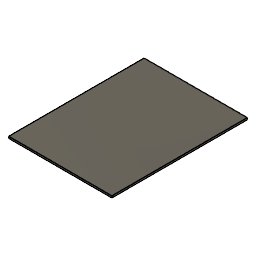
Maindarkprojectcomplete (Autodesk Fusion 360 archive; units mm, degrees)
design "pcb sketch"
part number: 2026-03-12-08-39-27-910
Autodesk Fusion 360 part; units mm, degrees
sketch "Sketch1" plane through (0, 0, 0) normal (0, 0, 1) x (1, 0, 0)
  line L0 (-24.7329, 57.4075) -> (32.4171, 57.4075)
  line L1 (32.4171, 57.4075) -> (32.4171, -17.5925)
  line L2 (32.4171, -17.5925) -> (-24.7329, -17.5925)
  line L3 (-24.7329, -17.5925) -> (-24.7329, 57.4075)
  dimension "d1" = 57.15
  dimension "d2" = 75
  constraint horizontal L0
  constraint vertical L1
  constraint horizontal L2
  constraint vertical L3
  measures "d1" distance of L0.start L0.end
  measures "d2" distance of L0 L2
extrude "Extrude1" add sketch "Sketch1" along normal blind 1

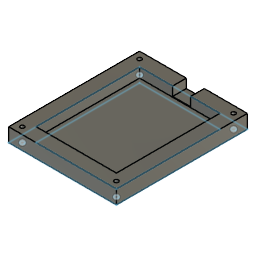
design "Darckprojectbottom"
part number: 2026-03-10-08-40-41-572
Autodesk Fusion 360 part; units mm, degrees
sketch "Sketch1" plane through (0, 0, 0) normal (0, 0, 1) x (1, 0, 0)
  line L0 (-50, 50) -> (8.2, 50)
  line L1 (8.2, 50) -> (8.2, -25)
  line L2 (8.2, -25) -> (-50, -25)
  line L3 (-50, -25) -> (-50, 50)
  line L4 (-60, 60) -> (18.2, 60)
  line L5 (18.2, 60) -> (18.2, -35)
  line L6 (18.2, -35) -> (-60, -35)
  line L7 (-60, -35) -> (-60, 60)
  circle A0 centre (-55, 55) radius 1.45
  circle A1 centre (13.2, 55) radius 1.45
  circle A2 centre (-55, -30) radius 1.45
  circle A3 centre (13.2, -30) radius 1.45
  dimension "d1" = 58.2
  dimension "d2" = 75
  dimension "d3" = 10
  dimension "d4" = 10
  dimension "d5" = 10
  dimension "d6" = 10
  dimension "d13" = 2.9
  dimension "d14" = 5
  dimension "d15" = 5
  dimension "d16" = 2.9
  dimension "d17" = 5
  dimension "d18" = 5
  dimension "d19" = 2.9
  dimension "d20" = 5
  dimension "d21" = 5
  dimension "d22" = 2.9
  dimension "d23" = 5
  dimension "d24" = 5
  constraint horizontal L0
  constraint vertical L1
  constraint horizontal L2
  constraint vertical L3
  constraint horizontal L4
  constraint vertical L5
  constraint horizontal L6
  constraint vertical L7
  measures "d1" distance of L0.start L0.end
  measures "d2" distance of L0 L2
  measures "d3" distance of L0 L4
  measures "d4" distance of L1 L5
  measures "d5" distance of L2 L6
  measures "d6" distance of L3 L7
  measures "d13" diameter of A0
  measures "d14" distance of L7 A0.centre
  measures "d15" distance of L4 A0.centre
  measures "d16" diameter of A1
  measures "d17" distance of L5 A1.centre
  measures "d18" distance of L4 A1.centre
  measures "d19" diameter of A2
  measures "d20" distance of L7 A2.centre
  measures "d21" distance of L6 A2.centre
  measures "d22" diameter of A3
  measures "d23" distance of L5 A3.centre
  measures "d24" distance of L6 A3.centre
sketch "Sketch3" plane through (0, 60, 0) normal (0, 1, 0) x (-1, 0, 0)
  line L0 (-17.15, 3) -> (60, 3)
  line L1 (60, 3) -> (60, 13)
  line L2 (60, 13) -> (-17.15, 13)
  line L3 (-17.15, 13) -> (-17.15, 3)
  line L4 (13.06, 13.5) -> (26.06, 13.5)
  line L5 (26.06, 13.5) -> (26.06, 3.5)
  line L6 (26.06, 3.5) -> (13.06, 3.5)
  line L7 (13.06, 3.5) -> (13.06, 13.5)
  dimension "d30" = 13
  dimension "d31" = 10
  dimension "d32" = 0.5
  dimension "d33" = 33.94
  constraint horizontal L4
  constraint vertical L5
  constraint horizontal L6
  constraint vertical L7
  measures "d30" distance of L4.start L4.end
  measures "d31" distance of L4 L6
  measures "d32" distance of L0 L6
  measures "d33" distance of L1 L5
extrude "Extrude7" add sketch "Sketch1" along normal blind 3 contours L0 L1 L2 L3 | L4 L5 L6 L7
extrude "Extrude8" add sketch "Sketch1" along normal blind 10
extrude "Extrude9" cut sketch "Sketch3" against normal blind 10 contours L2 L5 L6 L7

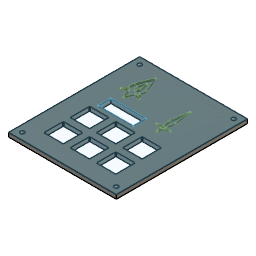
design "Darkprojectcaseupper"
part number: 2026-03-10-08-39-43-669
Autodesk Fusion 360 part; units mm, degrees
sketch "Sketch1" plane through (0, 0, 0) normal (0, 0, 1) x (1, 0, 0)
  line L0 (-36.5321, 51.7348) -> (21.6679, 51.7348)
  line L1 (21.6679, 51.7348) -> (21.6679, -23.2652)
  line L2 (21.6679, -23.2652) -> (-36.5321, -23.2652)
  line L3 (-36.5321, -23.2652) -> (-36.5321, 51.7348)
  line L4 (-46.5321, 61.894) -> (31.6679, 61.894)
  line L5 (31.6679, 61.894) -> (31.6679, -33.2652)
  line L6 (31.6679, -33.2652) -> (-46.5321, -33.2652)
  line L7 (-46.5321, -33.2652) -> (-46.5321, 61.894)
  circle A0 centre (-41.5321, -28.2652) radius 1.45
  circle A1 centre (26.6679, -28.2652) radius 1.45
  circle A2 centre (26.6679, 56.894) radius 1.45
  circle A3 centre (-41.5321, 56.894) radius 1.45
  dimension "d1" = 58.2
  dimension "d2" = 75
  dimension "d3" = 78.2
  dimension "d4" = 10
  dimension "d5" = 10
  dimension "d6" = 2.9
  dimension "d7" = 5
  dimension "d8" = 5
  dimension "d9" = 2.9
  dimension "d10" = 5
  dimension "d11" = 5
  dimension "d12" = 2.9
  dimension "d13" = 5
  dimension "d14" = 5
  dimension "d15" = 2.9
  dimension "d16" = 5
  dimension "d17" = 5
  constraint horizontal L0
  constraint vertical L1
  constraint horizontal L2
  constraint vertical L3
  constraint horizontal L4
  constraint vertical L5
  constraint horizontal L6
  constraint vertical L7
  measures "d1" distance of L0.start L0.end
  measures "d2" distance of L0 L2
  measures "d3" distance of L4.start L4.end
  measures "d4" distance of L1 L5
  measures "d5" distance of L2 L6
  measures "d6" diameter of A0
  measures "d7" distance of L6 A0.centre
  measures "d8" distance of L7 A0.centre
  measures "d9" diameter of A1
  measures "d10" distance of L5 A1.centre
  measures "d11" distance of L6 A1.centre
  measures "d12" diameter of A2
  measures "d13" distance of L5 A2.centre
  measures "d14" distance of L4 A2.centre
  measures "d15" diameter of A3
  measures "d16" distance of L4 A3.centre
  measures "d17" distance of L7 A3.centre
extrude "Extrude1" add sketch "Sketch1" along normal blind 3 contours L0 L1 L2 L3 | L4 L5 L6 L7
sketch "plate-2026-03-10T08_09_48.160Z" plane through (0, 0, 3) normal (0, 0, 1) x (1, 0, 0)
  line L0 (-13.925, 12.475) -> (-0.925, 12.475)
  line L1 (-13.925, -1.525) -> (-0.925, -1.525)
  line L2 (-14.425, 11.975) -> (-14.425, -1.025)
  line L3 (-0.425, 11.975) -> (-0.425, -1.025)
  arc A0 (-13.925, 12.475) -> (-14.425, 11.975) centre (-13.925, 11.975) ccw
  arc A1 (-0.425, 11.975) -> (-0.925, 12.475) centre (-0.925, 11.975) ccw
  arc A2 (-14.425, -1.025) -> (-13.925, -1.525) centre (-13.925, -1.025) ccw
  arc A3 (-0.925, -1.525) -> (-0.425, -1.025) centre (-0.925, -1.025) ccw
  line L4 (5.125, 12.475) -> (18.125, 12.475)
  line L5 (5.125, -1.525) -> (18.125, -1.525)
  line L6 (4.625, 11.975) -> (4.625, -1.025)
  line L7 (18.625, 11.975) -> (18.625, -1.025)
  arc A4 (5.125, 12.475) -> (4.625, 11.975) centre (5.125, 11.975) ccw
  arc A5 (18.625, 11.975) -> (18.125, 12.475) centre (18.125, 11.975) ccw
  arc A6 (4.625, -1.025) -> (5.125, -1.525) centre (5.125, -1.025) ccw
  arc A7 (18.125, -1.525) -> (18.625, -1.025) centre (18.125, -1.025) ccw
  line L8 (-32.975, -6.575) -> (-19.975, -6.575)
  line L9 (-32.975, -20.575) -> (-19.975, -20.575)
  line L10 (-33.475, -7.075) -> (-33.475, -20.075)
  line L11 (-19.475, -7.075) -> (-19.475, -20.075)
  arc A8 (-32.975, -6.575) -> (-33.475, -7.075) centre (-32.975, -7.075) ccw
  arc A9 (-19.475, -7.075) -> (-19.975, -6.575) centre (-19.975, -7.075) ccw
  arc A10 (-33.475, -20.075) -> (-32.975, -20.575) centre (-32.975, -20.075) ccw
  arc A11 (-19.975, -20.575) -> (-19.475, -20.075) centre (-19.975, -20.075) ccw
  line L12 (-13.925, -6.575) -> (-0.925, -6.575)
  line L13 (-13.925, -20.575) -> (-0.925, -20.575)
  line L14 (-14.425, -7.075) -> (-14.425, -20.075)
  line L15 (-0.425, -7.075) -> (-0.425, -20.075)
  arc A12 (-13.925, -6.575) -> (-14.425, -7.075) centre (-13.925, -7.075) ccw
  arc A13 (-0.425, -7.075) -> (-0.925, -6.575) centre (-0.925, -7.075) ccw
  arc A14 (-14.425, -20.075) -> (-13.925, -20.575) centre (-13.925, -20.075) ccw
  arc A15 (-0.925, -20.575) -> (-0.425, -20.075) centre (-0.925, -20.075) ccw
  line L16 (5.125, -6.575) -> (18.125, -6.575)
  line L17 (5.125, -20.575) -> (18.125, -20.575)
  line L18 (4.625, -7.075) -> (4.625, -20.075)
  line L19 (18.625, -7.075) -> (18.625, -20.075)
  arc A16 (5.125, -6.575) -> (4.625, -7.075) centre (5.125, -7.075) ccw
  arc A17 (18.625, -7.075) -> (18.125, -6.575) centre (18.125, -7.075) ccw
  arc A18 (4.625, -20.075) -> (5.125, -20.575) centre (5.125, -20.075) ccw
  arc A19 (18.125, -20.575) -> (18.625, -20.075) centre (18.125, -20.075) ccw
  line L20 (-36, -23.1) -> (21.15, -23.1)
  line L21 (-36, 15) -> (21.15, 15)
  line L22 (-36, -23.1) -> (-36, 15)
  line L23 (21.15, -23.1) -> (21.15, 15)
extrude "Extrude2" cut sketch "plate-2026-03-10T08_09_48.160Z" against normal blind 3 contours L0 L1 L2 L3 A0 A1 A2 A3 | L4 L5 L6 L7 A4 A5 A6 A7 | L8 L9 L10 L11 A8 A9 A10 A11 | L12 L13 L14 L15 A12 A13 A14 A15 | L16 L17 L18 L19 A16 A17 A18 A19
sketch "plate-2026-03-10T20_02_18.026Z" plane through (0, 0, 3) normal (0, 0, 1) x (1, 0, 0)
  line L0 (-32.975, 12.475) -> (-19.975, 12.475)
  line L1 (-32.975, -1.525) -> (-19.975, -1.525)
  line L2 (-33.475, 11.975) -> (-33.475, -1.025)
  line L3 (-19.475, 11.975) -> (-19.475, -1.025)
  arc A0 (-32.975, 12.475) -> (-33.475, 11.975) centre (-32.975, 11.975) ccw
  arc A1 (-19.475, 11.975) -> (-19.975, 12.475) centre (-19.975, 11.975) ccw
  arc A2 (-33.475, -1.025) -> (-32.975, -1.525) centre (-32.975, -1.025) ccw
  arc A3 (-19.975, -1.525) -> (-19.475, -1.025) centre (-19.975, -1.025) ccw
  line L4 (-13.925, 12.475) -> (-0.925, 12.475)
  line L5 (-13.925, -1.525) -> (-0.925, -1.525)
  line L6 (-14.425, 11.975) -> (-14.425, -1.025)
  line L7 (-0.425, 11.975) -> (-0.425, -1.025)
  arc A4 (-13.925, 12.475) -> (-14.425, 11.975) centre (-13.925, 11.975) ccw
  arc A5 (-0.425, 11.975) -> (-0.925, 12.475) centre (-0.925, 11.975) ccw
  arc A6 (-14.425, -1.025) -> (-13.925, -1.525) centre (-13.925, -1.025) ccw
  arc A7 (-0.925, -1.525) -> (-0.425, -1.025) centre (-0.925, -1.025) ccw
  line L8 (5.125, 12.475) -> (18.125, 12.475)
  line L9 (5.125, -1.525) -> (18.125, -1.525)
  line L10 (4.625, 11.975) -> (4.625, -1.025)
  line L11 (18.625, 11.975) -> (18.625, -1.025)
  arc A8 (5.125, 12.475) -> (4.625, 11.975) centre (5.125, 11.975) ccw
  arc A9 (18.625, 11.975) -> (18.125, 12.475) centre (18.125, 11.975) ccw
  arc A10 (4.625, -1.025) -> (5.125, -1.525) centre (5.125, -1.025) ccw
  arc A11 (18.125, -1.525) -> (18.625, -1.025) centre (18.125, -1.025) ccw
  line L12 (-32.975, -6.575) -> (-19.975, -6.575)
  line L13 (-32.975, -20.575) -> (-19.975, -20.575)
  line L14 (-33.475, -7.075) -> (-33.475, -20.075)
  line L15 (-19.475, -7.075) -> (-19.475, -20.075)
  arc A12 (-32.975, -6.575) -> (-33.475, -7.075) centre (-32.975, -7.075) ccw
  arc A13 (-19.475, -7.075) -> (-19.975, -6.575) centre (-19.975, -7.075) ccw
  arc A14 (-33.475, -20.075) -> (-32.975, -20.575) centre (-32.975, -20.075) ccw
  arc A15 (-19.975, -20.575) -> (-19.475, -20.075) centre (-19.975, -20.075) ccw
  line L16 (-13.925, -6.575) -> (-0.925, -6.575)
  line L17 (-13.925, -20.575) -> (-0.925, -20.575)
  line L18 (-14.425, -7.075) -> (-14.425, -20.075)
  line L19 (-0.425, -7.075) -> (-0.425, -20.075)
  arc A16 (-13.925, -6.575) -> (-14.425, -7.075) centre (-13.925, -7.075) ccw
  arc A17 (-0.425, -7.075) -> (-0.925, -6.575) centre (-0.925, -7.075) ccw
  arc A18 (-14.425, -20.075) -> (-13.925, -20.575) centre (-13.925, -20.075) ccw
  arc A19 (-0.925, -20.575) -> (-0.425, -20.075) centre (-0.925, -20.075) ccw
  line L20 (5.125, -6.575) -> (18.125, -6.575)
  line L21 (5.125, -20.575) -> (18.125, -20.575)
  line L22 (4.625, -7.075) -> (4.625, -20.075)
  line L23 (18.625, -7.075) -> (18.625, -20.075)
  arc A20 (5.125, -6.575) -> (4.625, -7.075) centre (5.125, -7.075) ccw
  arc A21 (18.625, -7.075) -> (18.125, -6.575) centre (18.125, -7.075) ccw
  arc A22 (4.625, -20.075) -> (5.125, -20.575) centre (5.125, -20.075) ccw
  arc A23 (18.125, -20.575) -> (18.625, -20.075) centre (18.125, -20.075) ccw
  line L24 (-36, -23.1) -> (21.15, -23.1)
  line L25 (-36, 15) -> (21.15, 15)
  line L26 (-36, -23.1) -> (-36, 15)
  line L27 (21.15, -23.1) -> (21.15, 15)
extrude "Extrude3" cut sketch "plate-2026-03-10T20_02_18.026Z" against normal blind 3 contours L0 L1 L2 L3 A0 A1 A2 A3
sketch "Sketch6" plane through (0, 0, 3) normal (0, 0, 1) x (-1, 0, 0)
  line L0 (33.475, 1.025) -> (33.475, -11.975)
  arc A0 (32.975, -12.475) -> (33.475, -11.975) centre (32.975, -11.975) ccw
  line L1 (32.975, -12.475) -> (19.975, -12.475)
  arc A1 (19.475, -11.975) -> (19.975, -12.475) centre (19.975, -11.975) ccw
  line L2 (19.475, -11.975) -> (19.475, 1.025)
  arc A2 (19.975, 1.525) -> (19.475, 1.025) centre (19.975, 1.025) ccw
  line L3 (19.975, 1.525) -> (32.975, 1.525)
  arc A3 (33.475, 1.025) -> (32.975, 1.525) centre (32.975, 1.025) ccw
  line L4 (-4.625, 20.075) -> (-4.625, 7.075)
  arc A4 (-5.125, 6.575) -> (-4.625, 7.075) centre (-5.125, 7.075) ccw
  line L5 (-5.125, 6.575) -> (-18.125, 6.575)
  arc A5 (-18.625, 7.075) -> (-18.125, 6.575) centre (-18.125, 7.075) ccw
  line L6 (-18.625, 7.075) -> (-18.625, 20.075)
  arc A6 (-18.125, 20.575) -> (-18.625, 20.075) centre (-18.125, 20.075) ccw
  line L7 (-18.125, 20.575) -> (-5.125, 20.575)
  arc A7 (-4.625, 20.075) -> (-5.125, 20.575) centre (-5.125, 20.075) ccw
  line L8 (-4.625, 1.025) -> (-4.625, -11.975)
  arc A8 (-5.125, -12.475) -> (-4.625, -11.975) centre (-5.125, -11.975) ccw
  line L9 (-5.125, -12.475) -> (-18.125, -12.475)
  arc A9 (-18.625, -11.975) -> (-18.125, -12.475) centre (-18.125, -11.975) ccw
  line L10 (-18.625, -11.975) -> (-18.625, 1.025)
  arc A10 (-18.125, 1.525) -> (-18.625, 1.025) centre (-18.125, 1.025) ccw
  line L11 (-18.125, 1.525) -> (-5.125, 1.525)
  arc A11 (-4.625, 1.025) -> (-5.125, 1.525) centre (-5.125, 1.025) ccw
  line L12 (14.425, 20.075) -> (14.425, 7.075)
  arc A12 (13.925, 6.575) -> (14.425, 7.075) centre (13.925, 7.075) ccw
  line L13 (13.925, 6.575) -> (0.925, 6.575)
  arc A13 (0.425, 7.075) -> (0.925, 6.575) centre (0.925, 7.075) ccw
  line L14 (0.425, 7.075) -> (0.425, 20.075)
  arc A14 (0.925, 20.575) -> (0.425, 20.075) centre (0.925, 20.075) ccw
  line L15 (0.925, 20.575) -> (13.925, 20.575)
  arc A15 (14.425, 20.075) -> (13.925, 20.575) centre (13.925, 20.075) ccw
  line L16 (14.425, 1.025) -> (14.425, -11.975)
  arc A16 (13.925, -12.475) -> (14.425, -11.975) centre (13.925, -11.975) ccw
  line L17 (13.925, -12.475) -> (0.925, -12.475)
  arc A17 (0.425, -11.975) -> (0.925, -12.475) centre (0.925, -11.975) ccw
  line L18 (0.425, -11.975) -> (0.425, 1.025)
  arc A18 (0.925, 1.525) -> (0.425, 1.025) centre (0.925, 1.025) ccw
  line L19 (0.925, 1.525) -> (13.925, 1.525)
  arc A19 (14.425, 1.025) -> (13.925, 1.525) centre (13.925, 1.025) ccw
  line L20 (33.475, 20.075) -> (33.475, 7.075)
  arc A20 (32.975, 6.575) -> (33.475, 7.075) centre (32.975, 7.075) ccw
  line L21 (32.975, 6.575) -> (19.975, 6.575)
  arc A21 (19.475, 7.075) -> (19.975, 6.575) centre (19.975, 7.075) ccw
  line L22 (19.475, 7.075) -> (19.475, 20.075)
  arc A22 (19.975, 20.575) -> (19.475, 20.075) centre (19.975, 20.075) ccw
  line L23 (19.975, 20.575) -> (32.975, 20.575)
  arc A23 (33.475, 20.075) -> (32.975, 20.575) centre (32.975, 20.075) ccw
  circle A24 centre (-26.6679, 28.2652) radius 1.45
  circle A25 centre (41.5321, -56.894) radius 1.45
  circle A26 centre (41.5321, 28.2652) radius 1.45
  circle A27 centre (-26.6679, -56.894) radius 1.45
  line L24 (46.5321, 33.2652) -> (-31.6679, 33.2652)
  line L25 (-31.6679, 33.2652) -> (-31.6679, -61.894)
  line L26 (-31.6679, -61.894) -> (46.5321, -61.894)
  line L27 (46.5321, -61.894) -> (46.5321, 33.2652)
  line L28 (30.5252, -25) -> (5.2252, -25)
  line L29 (5.2252, -25) -> (5.2252, -15.9341)
  line L30 (5.2252, -15.9341) -> (30.5252, -15.9341)
  line L31 (30.5252, -15.9341) -> (30.5252, -25)
  dimension "d28" = 25.3
  constraint horizontal L28
  constraint vertical L29
  constraint horizontal L30
  constraint vertical L31
  measures "d28" distance of L28.start L28.end
extrude "Extrude5" cut sketch "Sketch6" against normal blind 3 contours L28 L29 L30 L31
sketch "Sketch7" plane through (0, 0, 3) normal (0, 0, 1) x (-1, 0, 0)
  line L0 (5.2252, -25) -> (5.2252, -15.9341)
  line L1 (5.2252, -15.9341) -> (30.5252, -15.9341)
  line L2 (30.5252, -15.9341) -> (30.5252, -25)
  line L3 (30.5252, -25) -> (5.2252, -25)
  line L4 (33.475, 1.025) -> (33.475, -11.975)
  arc A0 (32.975, -12.475) -> (33.475, -11.975) centre (32.975, -11.975) ccw
  line L5 (32.975, -12.475) -> (19.975, -12.475)
  arc A1 (19.475, -11.975) -> (19.975, -12.475) centre (19.975, -11.975) ccw
  line L6 (19.475, -11.975) -> (19.475, 1.025)
  arc A2 (19.975, 1.525) -> (19.475, 1.025) centre (19.975, 1.025) ccw
  line L7 (19.975, 1.525) -> (32.975, 1.525)
  arc A3 (33.475, 1.025) -> (32.975, 1.525) centre (32.975, 1.025) ccw
  line L8 (-4.625, 20.075) -> (-4.625, 7.075)
  arc A4 (-5.125, 6.575) -> (-4.625, 7.075) centre (-5.125, 7.075) ccw
  line L9 (-5.125, 6.575) -> (-18.125, 6.575)
  arc A5 (-18.625, 7.075) -> (-18.125, 6.575) centre (-18.125, 7.075) ccw
  line L10 (-18.625, 7.075) -> (-18.625, 20.075)
  arc A6 (-18.125, 20.575) -> (-18.625, 20.075) centre (-18.125, 20.075) ccw
  line L11 (-18.125, 20.575) -> (-5.125, 20.575)
  arc A7 (-4.625, 20.075) -> (-5.125, 20.575) centre (-5.125, 20.075) ccw
  line L12 (-4.625, 1.025) -> (-4.625, -11.975)
  arc A8 (-5.125, -12.475) -> (-4.625, -11.975) centre (-5.125, -11.975) ccw
  line L13 (-5.125, -12.475) -> (-18.125, -12.475)
  arc A9 (-18.625, -11.975) -> (-18.125, -12.475) centre (-18.125, -11.975) ccw
  line L14 (-18.625, -11.975) -> (-18.625, 1.025)
  arc A10 (-18.125, 1.525) -> (-18.625, 1.025) centre (-18.125, 1.025) ccw
  line L15 (-18.125, 1.525) -> (-5.125, 1.525)
  arc A11 (-4.625, 1.025) -> (-5.125, 1.525) centre (-5.125, 1.025) ccw
  line L16 (14.425, 20.075) -> (14.425, 7.075)
  arc A12 (13.925, 6.575) -> (14.425, 7.075) centre (13.925, 7.075) ccw
  line L17 (13.925, 6.575) -> (0.925, 6.575)
  arc A13 (0.425, 7.075) -> (0.925, 6.575) centre (0.925, 7.075) ccw
  line L18 (0.425, 7.075) -> (0.425, 20.075)
  arc A14 (0.925, 20.575) -> (0.425, 20.075) centre (0.925, 20.075) ccw
  line L19 (0.925, 20.575) -> (13.925, 20.575)
  arc A15 (14.425, 20.075) -> (13.925, 20.575) centre (13.925, 20.075) ccw
  line L20 (14.425, 1.025) -> (14.425, -11.975)
  arc A16 (13.925, -12.475) -> (14.425, -11.975) centre (13.925, -11.975) ccw
  line L21 (13.925, -12.475) -> (0.925, -12.475)
  arc A17 (0.425, -11.975) -> (0.925, -12.475) centre (0.925, -11.975) ccw
  line L22 (0.425, -11.975) -> (0.425, 1.025)
  arc A18 (0.925, 1.525) -> (0.425, 1.025) centre (0.925, 1.025) ccw
  line L23 (0.925, 1.525) -> (13.925, 1.525)
  arc A19 (14.425, 1.025) -> (13.925, 1.525) centre (13.925, 1.025) ccw
  line L24 (33.475, 20.075) -> (33.475, 7.075)
  arc A20 (32.975, 6.575) -> (33.475, 7.075) centre (32.975, 7.075) ccw
  line L25 (32.975, 6.575) -> (19.975, 6.575)
  arc A21 (19.475, 7.075) -> (19.975, 6.575) centre (19.975, 7.075) ccw
  line L26 (19.475, 7.075) -> (19.475, 20.075)
  arc A22 (19.975, 20.575) -> (19.475, 20.075) centre (19.975, 20.075) ccw
  line L27 (19.975, 20.575) -> (32.975, 20.575)
  arc A23 (33.475, 20.075) -> (32.975, 20.575) centre (32.975, 20.075) ccw
  circle A24 centre (-26.6679, 28.2652) radius 1.45
  circle A25 centre (41.5321, -56.894) radius 1.45
  circle A26 centre (41.5321, 28.2652) radius 1.45
  circle A27 centre (-26.6679, -56.894) radius 1.45
  line L28 (46.5321, 33.2652) -> (-31.6679, 33.2652)
  line L29 (-31.6679, 33.2652) -> (-31.6679, -61.894)
  line L30 (-31.6679, -61.894) -> (46.5321, -61.894)
  line L31 (46.5321, -61.894) -> (46.5321, 33.2652)
  line L32 (-6.7708, -21.3229) -> (-5.7125, -24.7625)
  line L33 (-5.7125, -24.7625) -> (-2.0083, -25.8208)
  line L34 (-2.0083, -25.8208) -> (-5.7125, -26.8792)
  line L35 (-5.7125, -26.8792) -> (-4.9187, -32.7)
  line L36 (-4.9187, -32.7) -> (-6.7708, -45.1354)
  line L37 (-6.7708, -45.1354) -> (-8.6229, -32.7)
  line L38 (-8.6229, -32.7) -> (-7.8292, -26.8792)
  line L39 (-7.8292, -26.8792) -> (-11.5333, -25.8208)
  line L40 (-11.5333, -25.8208) -> (-7.8292, -24.7625)
  line L41 (-7.8292, -24.7625) -> (-6.7708, -21.3229)
extrude "Extrude6" cut sketch "Sketch7" against normal blind 0.5 contours L32 L33 L34 L35 L36 L37 L38 L39 L40 L41
sketch "Sketch8" plane through (0, 0, 3) normal (0, 0, 1) x (-1, 0, 0)
  line L0 (-7.8292, -26.8792) -> (-11.5333, -25.8208)
  line L1 (-11.5333, -25.8208) -> (-7.8292, -24.7625)
  line L2 (-7.8292, -24.7625) -> (-6.7708, -21.3229)
  line L3 (-6.7708, -21.3229) -> (-5.7125, -24.7625)
  line L4 (-5.7125, -24.7625) -> (-2.0083, -25.8208)
  line L5 (-2.0083, -25.8208) -> (-5.7125, -26.8792)
  line L6 (-5.7125, -26.8792) -> (-4.9187, -32.7)
  line L7 (-4.9187, -32.7) -> (-6.7708, -45.1354)
  line L8 (-6.7708, -45.1354) -> (-8.6229, -32.7)
  line L9 (-8.6229, -32.7) -> (-7.8292, -26.8792)
  line L10 (5.2252, -25) -> (5.2252, -15.9341)
  line L11 (5.2252, -15.9341) -> (30.5252, -15.9341)
  line L12 (30.5252, -15.9341) -> (30.5252, -25)
  line L13 (30.5252, -25) -> (5.2252, -25)
  line L14 (33.475, 1.025) -> (33.475, -11.975)
  arc A0 (32.975, -12.475) -> (33.475, -11.975) centre (32.975, -11.975) ccw
  line L15 (32.975, -12.475) -> (19.975, -12.475)
  arc A1 (19.475, -11.975) -> (19.975, -12.475) centre (19.975, -11.975) ccw
  line L16 (19.475, -11.975) -> (19.475, 1.025)
  arc A2 (19.975, 1.525) -> (19.475, 1.025) centre (19.975, 1.025) ccw
  line L17 (19.975, 1.525) -> (32.975, 1.525)
  arc A3 (33.475, 1.025) -> (32.975, 1.525) centre (32.975, 1.025) ccw
  line L18 (-4.625, 20.075) -> (-4.625, 7.075)
  arc A4 (-5.125, 6.575) -> (-4.625, 7.075) centre (-5.125, 7.075) ccw
  line L19 (-5.125, 6.575) -> (-18.125, 6.575)
  arc A5 (-18.625, 7.075) -> (-18.125, 6.575) centre (-18.125, 7.075) ccw
  line L20 (-18.625, 7.075) -> (-18.625, 20.075)
  arc A6 (-18.125, 20.575) -> (-18.625, 20.075) centre (-18.125, 20.075) ccw
  line L21 (-18.125, 20.575) -> (-5.125, 20.575)
  arc A7 (-4.625, 20.075) -> (-5.125, 20.575) centre (-5.125, 20.075) ccw
  line L22 (-4.625, 1.025) -> (-4.625, -11.975)
  arc A8 (-5.125, -12.475) -> (-4.625, -11.975) centre (-5.125, -11.975) ccw
  line L23 (-5.125, -12.475) -> (-18.125, -12.475)
  arc A9 (-18.625, -11.975) -> (-18.125, -12.475) centre (-18.125, -11.975) ccw
  line L24 (-18.625, -11.975) -> (-18.625, 1.025)
  arc A10 (-18.125, 1.525) -> (-18.625, 1.025) centre (-18.125, 1.025) ccw
  line L25 (-18.125, 1.525) -> (-5.125, 1.525)
  arc A11 (-4.625, 1.025) -> (-5.125, 1.525) centre (-5.125, 1.025) ccw
  line L26 (14.425, 20.075) -> (14.425, 7.075)
  arc A12 (13.925, 6.575) -> (14.425, 7.075) centre (13.925, 7.075) ccw
  line L27 (13.925, 6.575) -> (0.925, 6.575)
  arc A13 (0.425, 7.075) -> (0.925, 6.575) centre (0.925, 7.075) ccw
  line L28 (0.425, 7.075) -> (0.425, 20.075)
  arc A14 (0.925, 20.575) -> (0.425, 20.075) centre (0.925, 20.075) ccw
  line L29 (0.925, 20.575) -> (13.925, 20.575)
  arc A15 (14.425, 20.075) -> (13.925, 20.575) centre (13.925, 20.075) ccw
  line L30 (14.425, 1.025) -> (14.425, -11.975)
  arc A16 (13.925, -12.475) -> (14.425, -11.975) centre (13.925, -11.975) ccw
  line L31 (13.925, -12.475) -> (0.925, -12.475)
  arc A17 (0.425, -11.975) -> (0.925, -12.475) centre (0.925, -11.975) ccw
  line L32 (0.425, -11.975) -> (0.425, 1.025)
  arc A18 (0.925, 1.525) -> (0.425, 1.025) centre (0.925, 1.025) ccw
  line L33 (0.925, 1.525) -> (13.925, 1.525)
  arc A19 (14.425, 1.025) -> (13.925, 1.525) centre (13.925, 1.025) ccw
  line L34 (33.475, 20.075) -> (33.475, 7.075)
  arc A20 (32.975, 6.575) -> (33.475, 7.075) centre (32.975, 7.075) ccw
  line L35 (32.975, 6.575) -> (19.975, 6.575)
  arc A21 (19.475, 7.075) -> (19.975, 6.575) centre (19.975, 7.075) ccw
  line L36 (19.475, 7.075) -> (19.475, 20.075)
  arc A22 (19.975, 20.575) -> (19.475, 20.075) centre (19.975, 20.075) ccw
  line L37 (19.975, 20.575) -> (32.975, 20.575)
  arc A23 (33.475, 20.075) -> (32.975, 20.575) centre (32.975, 20.075) ccw
  circle A24 centre (-26.6679, 28.2652) radius 1.45
  circle A25 centre (41.5321, -56.894) radius 1.45
  circle A26 centre (41.5321, 28.2652) radius 1.45
  circle A27 centre (-26.6679, -56.894) radius 1.45
  line L38 (46.5321, 33.2652) -> (-31.6679, 33.2652)
  line L39 (-31.6679, 33.2652) -> (-31.6679, -61.894)
  line L40 (-31.6679, -61.894) -> (46.5321, -61.894)
  line L41 (46.5321, -61.894) -> (46.5321, 33.2652)
  spline S0 degree 3 poles (26.7708, -53.6771) (28.3583, -50.2375) (29.9458, -46.5333) (31.0042, -43.0937) knots 0 0 0 0 1 1 1 1
  spline S1 degree 3 poles (31.0042, -43.0937) (31.5333, -41.2417) (31.5333, -39.6542) (30.7396, -38.3312) knots 0 0 0 0 1 1 1 1
  line L42 (30.7396, -38.3312) -> (33.3854, -35.1562)
  line L43 (33.3854, -35.1562) -> (29.4167, -36.4792)
  spline S2 degree 3 poles (29.4167, -36.4792) (28.3583, -34.3625) (27.5646, -32.5104) (26.7708, -30.6583) knots 0 0 0 0 1 1 1 1
  spline S3 degree 3 poles (26.7708, -30.6583) (25.9771, -32.5104) (25.1833, -34.3625) (24.125, -36.4792) knots 0 0 0 0 1 1 1 1
  line L44 (24.125, -36.4792) -> (20.1563, -35.1562)
  line L45 (20.1563, -35.1562) -> (22.8021, -38.3312)
  spline S4 degree 3 poles (22.8021, -38.3312) (22.0083, -39.6542) (22.0083, -41.2417) (22.5375, -43.0937) knots 0 0 0 0 1 1 1 1
  spline S5 degree 3 poles (22.5375, -43.0937) (23.5958, -46.5333) (25.1833, -50.2375) (26.7708, -53.6771) knots 0 0 0 0 1 1 1 1
  spline S6 degree 3 poles (26.7708, -47.0625) (25.9771, -44.9458) (25.4479, -43.0937) (25.4479, -41.7708) knots 0 0 0 0 1 1 1 1
  spline S7 degree 3 poles (25.4479, -41.7708) (25.4479, -40.4479) (25.9771, -39.6542) (26.7708, -39.125) knots 0 0 0 0 1 1 1 1
  spline S8 degree 3 poles (26.7708, -39.125) (27.5646, -39.6542) (28.0938, -40.4479) (28.0938, -41.7708) knots 0 0 0 0 1 1 1 1
  spline S9 degree 3 poles (28.0938, -41.7708) (28.0938, -43.0937) (27.5646, -44.9458) (26.7708, -47.0625) knots 0 0 0 0 1 1 1 1
extrude "Extrude7" cut sketch "Sketch8" against normal blind 0.5 contours S0 S1 L42 L43 S2 S3 L44 L45 S4 S5

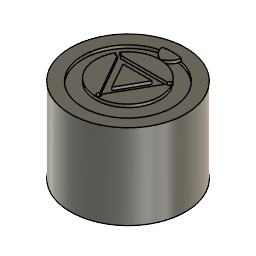
design "Untitled"
part number: 2026-03-13-09-33-52-471
Autodesk Fusion 360 part; units mm, degrees
sketch "Sketch1" plane through (0, 0, 0) normal (0, 0, 1) x (1, 0, 0)
  circle A0 centre (38.1204, 22.2369) radius 9.5
  dimension "d1" = 19
  measures "d1" diameter of A0
extrude "Extrude1" add sketch "Sketch1" along normal blind 14 makes body 1
sketch "Sketch3" plane through (0, 0, 0) normal (0, 0, 1) x (1, 0, 0)
  arc A0 (38.353, 24.7546) -> (40.7938, 22.3138) centre (38.353, 22.3138) cw
  arc A1 (40.7938, 22.3138) -> (38.353, 19.873) centre (38.353, 22.3138) cw
  line L0 (38.353, 19.873) -> (35.9122, 19.873)
  line L1 (35.9122, 19.873) -> (35.9122, 24.7546)
  line L2 (35.9122, 24.7546) -> (38.353, 24.7546)
extrude "Extrude2" cut sketch "Sketch3" along normal blind 10 bodies 1
sketch "Sketch4" plane through (0, 0, 14) normal (0, 0, 1) x (-1, 0, 0)
  circle A0 centre (-38.1204, -22.2369) radius 9.5
  circle A1 centre (-38.201, -22.1343) radius 7.4083
  circle A2 centre (-38.201, -22.1343) radius 5.2917
  line L0 (-38.201, -17.3718) -> (-33.9677, -24.7801)
  line L1 (-33.9677, -24.7801) -> (-42.4344, -24.7801)
  line L2 (-42.4344, -24.7801) -> (-38.201, -17.3718)
  line L3 (-38.201, -19.4884) -> (-35.8198, -23.7218)
  line L4 (-35.8198, -23.7218) -> (-40.5823, -23.7218)
  line L5 (-40.5823, -23.7218) -> (-38.201, -19.4884)
  line L6 (-38.201, -14.7259) -> (-38.201, -29.5426)
  line L7 (-45.6094, -22.1343) -> (-30.7927, -22.1343)
  line L8 (-40.8469, -16.3134) -> (-42.4344, -15.2551)
  line L9 (-35.5552, -16.3134) -> (-33.9677, -15.2551)
  spline S0 degree 3 poles (-38.201, -27.4259) (-37.1427, -27.9551) (-36.6135, -28.7488) (-36.6135, -29.5426) knots 0 0 0 0 1 1 1 1
  spline S1 degree 3 poles (-38.201, -27.4259) (-39.2594, -27.9551) (-39.7885, -28.7488) (-39.7885, -29.5426) knots 0 0 0 0 1 1 1 1
  circle A3 centre (-42.4344, -24.7801) radius 0.3704
  circle A4 centre (-33.9677, -24.7801) radius 0.3704
  circle A5 centre (-38.201, -17.3718) radius 0.3704
  point P0 (-32.9094, -22.1343)
  point P1 (-42.064, -24.7801)
  point P2 (-33.5973, -24.7801)
  point P3 (-37.8306, -17.3718)
extrude "Extrude3" cut sketch "Sketch4" against normal blind 0.5 contours A1 A2 L6 L7 | A1 A2 L7 S0 A4 | A1 L6 S0 | A2 L0 L6 L7 A5 | A2 L0 L7 A4 | A1 A2 L6 L7 | A1 L6 S1 | A1 A2 L7 S1 A3 | A2 L1 L6 A4 | A2 L1 L6 A3 | A2 L2 L6 L7 A5 | A2 A4 | A2 L0 L1 A4 | L0 L3 L6 L7 A5 | L0 L1 L3 L4 L6 L7 A4 | A2 A3 | A2 L1 L2 A3 | L1 L2 L4 L5 L6 L7 A3 | A2 L2 L7 A3 | L0 L6 A5 | L2 L6 A5 | L0 L1 A4 | L0 L6 A5 | L3 L6 L7 | L3 L4 L6 L7 | L1 L2 A3 | L4 L5 L6 L7 | L2 L5 L6 L7 A5 | L2 L6 A5 | L5 L6 L7 bodies 1
extrude "Extrude4" add sketch "Sketch4" along normal blind 0.5 separate body contours L3 L6 L7 | L3 L4 L6 L7 | L4 L5 L6 L7 | L5 L6 L7 makes body 2
extrude "Extrude5" add sketch "Sketch4" along normal blind 0.5 separate body contours A2 L0 L6 L7 A5 | A2 L0 L7 A4 | A2 L1 L6 A4 | A2 L1 L6 A3 | A2 L2 L6 L7 A5 | A2 L2 L7 A3 makes body 3 at (38.3325, 25.6571, 14) makes body 4 at (41.2514, 20.7773, 14.5)
extrude "Extrude6" add sketch "Sketch4" along normal blind 0.5 contours A1 L6 S0 | A1 L6 S1 bodies 1 3
